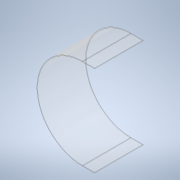
# Autodesk Inventor part: Glock Lexan
Saved by Autodesk Inventor 2020 (Build 240168000, 168)
## iProperties
Created: 2020-02-15
Part Number: Glock Lexan
Material: Polycarbonate, Clear
Document SubType Name: Modeling
Designer: aidan
Density: 1.2 g/cm^3
Appearance: Polycarbonate - Clear
Author: aidan
Autodesk Inventor part; units mm, degrees
ref_plane "YZ Plane" through (0, 0, 0) normal (1, 0, 0) x (0, 1, 0)
ref_plane "XZ Plane" through (0, 0, 0) normal (0, 1, 0) x (-1, 0, 0)
ref_plane "XY Plane" through (0, 0, 0) normal (0, 0, 1) x (1, 0, 0)
sketch "Sketch1" plane through (0, 0, 0) normal (1, 0, 0) x (0, 1, 0)
  line L0 (61.1429, 130.368) -> (58.1457, 130.368)
  line L1 (58.1457, 130.368) -> (58.1457, -72.832)
  line L2 (58.1457, -72.832) -> (61.1429, -72.832)
  line L3 (61.1429, -72.832) -> (61.1429, 130.368)
  line L4 (-129.3571, 80.0252) -> (-129.3571, -72.832) construction
  point P0 (0, 0)
  dimension "d0" = 2.9972
  dimension "d1" = 190.5
  dimension "d2" = 203.2
  constraints: 10 end point, 2 parallel, 1 horizontal, 1 perpendicular, 1 vertical
  measures "d0" distance between parallel lines of L1 L3
  measures "d1" distance between parallel lines of L4 L3
  measures "d2" distance of L2.end L0.start
revolve "Revolution1" add sketch "Sketch1" angle 180 about axis through (0, -129.3571, 80.0252) along (0, 0, 1)
sketch "Sketch2" plane through (0, 61.1429, 130.368) normal (1, 0, 0) x (0, 0, -1)
  line L0 (203.2, -2.9972) -> (203.2, 0) projected
  line L1 (203.2, 0) -> (0, 0) projected
  line L2 (0, 0) -> (0, -2.9972) projected
  line L3 (0, -2.9972) -> (203.2, -2.9972) projected
  line L4 (203.2, -381) -> (203.2, -378.0028) projected
  line L5 (203.2, -378.0028) -> (0, -378.0028) projected
  line L6 (0, -378.0028) -> (0, -381) projected
  line L7 (0, -381) -> (203.2, -381) projected
  point P0 (130.368, -61.1429)
extrude "Extrusion1" add sketch "Sketch2" along normal blind 50.8
body "Solid1"
